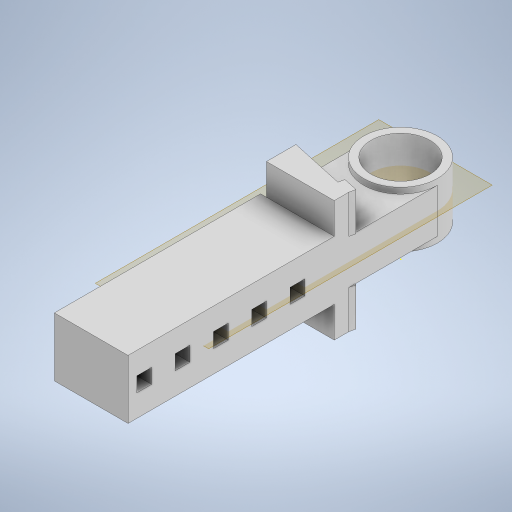
# Autodesk Inventor part: Part10copycopy
Saved by Autodesk Inventor 2023 (Build 270158000, 158)
## iProperties
Created: 2024-11-26
Part Number: Part10copycopy
Material: Generic
Document SubType Name: Modeling
Designer: 1ZHUSAM
Density: 1 g/cm^3
Appearance: Default
Author: 1ZHUSAM
Autodesk Inventor part; units mm, degrees
ref_plane "YZ Plane" through (0, 0, 0) normal (1, 0, 0) x (0, 1, 0)
ref_plane "XY Plane" through (0, 0, 0) normal (0, 0, 1) x (1, 0, 0)
sketch "Sketch1" plane through (0, 0, 0) normal (0, 1, 0) x (-1, 0, 0)
  circle A0 centre (0, 0) radius 10
  circle A1 centre (0, 0) radius 12.5
  line L0 (12.5, 0) -> (12.5, 50)
  line L1 (-12.5, 0) -> (-12.5, 50)
  line L2 (-12.5, 50) -> (12.5, 50)
  dimension "d0" = 20
  dimension "d1" = 25
  dimension "d2" = 50
  constraints: 6 end point, 2 centre point, 2 coincident, 2 point on circle, 2 tangent, 2 vertical, 1 perpendicular
  measures "d0" diameter of A0
  measures "d1" diameter of A1
  measures "d2" distance of L0.start L0.end
extrude "Extrusion1" add sketch "Sketch1" along normal blind 15
sketch "Sketch3" plane through (-12.5, 0, 50) normal (0, 0, 1) x (1, 0, 0)
  point P0 (12.5, 0)
sketch "Sketch4" plane through (-12.5, 0, 50) normal (0, 0, 1) x (1, 0, 0)
  line L0 (25, 0) -> (25, 15) projected
  line L1 (25, 0) -> (25, 15)
  line L2 (0, 15) -> (25, 15) projected
  line L3 (25, 15) -> (0, 15)
  line L4 (0, 0) -> (0, 15) projected
  line L5 (0, 15) -> (0, 0)
  line L6 (0, 0) -> (25, 0) projected
  line L7 (0, 0) -> (25, 0)
  point P0 (12.5, 0)
  constraints: 8 end point, 4 collinear
extrude "Extrusion3" add sketch "Sketch4" along normal blind 25
sketch "Sketch9" plane through (0, 0, 0) normal (0, -1, 0) x (1, 0, 0)
  line L0 (-12.5, 25) -> (-22.5, 25) projected
  line L1 (-12.5, 25) -> (12.5, 25)
  line L2 (12.5, 0) -> (12.5, 75) projected
  line L3 (-12.5, 25) -> (-12.5, 75) projected
  line L4 (-12.5, 25) -> (-12.5, 75)
  line L5 (-12.5, 75) -> (12.5, 75) projected
  line L6 (-12.5, 75) -> (12.5, 75)
  line L7 (12.5, 75) -> (12.5, 25)
  line L8 (12.5, 0) -> (12.5, 30)
  line L9 (-12.5, 25) -> (-10.5, 25)
  line L10 (-10.5, 25) -> (-10.5, 75)
  line L11 (-12.5, 75) -> (-12.5, 25)
  line L12 (-10.5, 25) -> (12.5, 30)
  line L13 (-10.5, 25) -> (-10.5, 35)
  line L14 (-10.5, 35) -> (12.5, 35)
  point P0 (0, 0)
  point P1 (12.5, 35)
  dimension "d50" = 30
  dimension "d51" = 2
  dimension "d74" = 10
  constraints: 22 end point, 7 point on line, 3 collinear, 3 perpendicular, 1 horizontal
  measures "d50" distance of L8.start L8.end
  measures "d51" distance of L0.start L9.end
  measures "d74" distance of L9.end L13.end
extrude "Extrusion7" add sketch "Sketch9" along normal blind 13 contours L10 L14 L2 L12
sketch "Sketch10" plane through (0, -13, 0) normal (0, -1, 0) x (1, 0, 0)
  point P0 (0, 0)
ref_plane "Work Plane1" through (0, 7.5, 0) normal (0, 1, 0) x (-1, 0, 0)
mirror "Mirror1" about plane through (0, 7.5, 0) normal (0, 1, 0) of "Extrusion7"
sketch "Sketch15" plane through (-10.5, 15, 25) normal (0.2124296, 0, -0.9771764) x (-0.9771764, 0, -0.2124296)
  line L0 (-23.5372, 0) -> (-23.5372, 13) projected
  line L1 (-14.7001, 13) -> (-18.6088, 13) projected
  line L2 (-23.5372, 0) -> (-18.5372, 0)
  line L3 (-18.5372, 0) -> (-18.5372, 13)
  line L4 (-18.5372, 13) -> (-23.5372, 13)
  line L5 (-23.5372, 13) -> (-23.5372, 0)
  line L6 (-23.5372, -28) -> (-24.5994, -28) projected
  line L7 (-18.6088, -28) -> (-18.6088, 13) projected
  line L8 (-23.5372, -28) -> (-18.6088, -28)
  line L9 (-18.6088, -28) -> (-18.6088, -15)
  line L10 (-18.6088, -15) -> (-23.5372, -15)
  line L11 (-23.5372, -15) -> (-23.5372, -28)
  point P0 (-4.9496, -15)
  point P1 (-33.0965, -28)
  point P2 (-18.6088, 0)
  point P3 (-23.5372, 13)
  dimension "d66" = 5
  constraints: 16 end point, 4 parallel, 2 horizontal, 2 perpendicular, 2 point on line
  measures "d66" distance of L4.end L3.end
extrude "Extrusion9" add sketch "Sketch15" along normal blind 2 contours L0 L4 L7 L2 | L8 L11 L10 L7
sketch "Sketch16" plane through (0, 15, 0) normal (0, 1, 0) x (1, 0, 0)
  circle A0 centre (0, 0) radius 10
  circle A1 centre (0, 0) radius 12.5
  dimension "d69" = 25
  constraints: 2 centre point, 2 coincident
  measures "d69" diameter of A1
extrude "Extrusion10" add sketch "Sketch16" along normal blind 2
sketch "Sketch17" plane through (0, 0, 0) normal (0, -1, 0) x (1, 0, 0)
  circle A0 centre (0, 0) radius 10
  circle A1 centre (0, 0) radius 10 projected
  circle A2 centre (0, 0) radius 12.5
  constraints: 2 centre point, 2 coincident
extrude "Extrusion11" add sketch "Sketch17" along normal blind 2
sketch "Sketch18" plane through (-12.5, 0, 0) normal (-1, 0, 0) x (0, 0, 1)
  point P0 (0, 0)
sketch "Sketch19" plane through (0, 0, 0) normal (0, -1, 0) x (1, 0, 0)
  line L0 (-12.5, 75) -> (12.5, 75) projected
  line L1 (12.5, 35) -> (-10.5, 35) projected
  line L2 (-12.5, 75) -> (12.5, 75)
  line L3 (12.5, 75) -> (12.5, 35)
  line L4 (12.5, 35) -> (-12.5, 35)
  line L5 (-12.5, 35) -> (-12.5, 75)
  point P0 (0, 0)
  constraints: 8 end point, 2 parallel, 1 horizontal, 1 perpendicular
extrude "Extrusion12" add sketch "Sketch19" along normal blind 2.5
sketch "Sketch20" plane through (0, 15, 0) normal (0, 1, 0) x (1, 0, 0)
  line L0 (12.5, -75) -> (-12.5, -75) projected
  line L1 (12.5, -35) -> (12.5, -75) projected
  line L2 (-12.5, -75) -> (12.5, -75)
  line L3 (12.5, -75) -> (12.5, -35)
  line L4 (12.5, -35) -> (-12.5, -35)
  line L5 (-12.5, -35) -> (-12.5, -75)
  point P0 (0, 0)
  constraints: 8 end point, 2 parallel, 1 horizontal, 1 perpendicular
extrude "Extrusion13" add sketch "Sketch20" along normal blind 2.5
sketch "Sketch21" plane through (-12.5, 0, 75) normal (0, 0, 1) x (1, 0, 0)
  line L0 (25, -2.5) -> (0, -2.5) projected
  line L1 (0, -2.5) -> (25, -2.5)
  line L2 (25, -2.5) -> (25, 17.5)
  line L3 (25, 17.5) -> (0, 17.5)
  line L4 (0, 17.5) -> (0, -2.5)
  point P0 (12.5, 0)
  constraints: 8 end point, 2 parallel, 1 horizontal, 1 perpendicular
extrude "Extrusion14" add sketch "Sketch21" along normal blind 30
sketch "Sketch22" plane through (-12.5, 0, 0) normal (-1, 0, 0) x (0, 0, 1)
  line L0 (35, 15) -> (35, 17.5) projected
  line L1 (35, -2.5) -> (105, -2.5) projected
  line L2 (35, 17.5) -> (45, 17.5)
  line L3 (45, 17.5) -> (45, -2.5)
  line L4 (45, -2.5) -> (35, -2.5)
  line L5 (35, -2.5) -> (35, 17.5)
  line L6 (45, 7.5) -> (50, 7.5)
  line L7 (45, 5) -> (50, 5)
  line L8 (50, 5) -> (50, 10)
  line L9 (50, 10) -> (45, 10)
  line L10 (45, 10) -> (45, 5)
  line L11 (45, 5) -> (50, 10) construction
  line L12 (50, 5) -> (45, 10) construction
  line L13 (50, 7.5) -> (58, 7.5)
  line L14 (63, 5) -> (58, 5)
  line L15 (58, 5) -> (58, 10)
  line L16 (58, 10) -> (63, 10)
  line L17 (63, 10) -> (63, 5)
  line L18 (63, 5) -> (58, 10) construction
  line L19 (58, 5) -> (63, 10) construction
  line L20 (63, 7.5) -> (71, 7.5)
  line L21 (76, 5) -> (71, 5)
  line L22 (71, 5) -> (71, 10)
  line L23 (71, 10) -> (76, 10)
  line L24 (76, 10) -> (76, 5)
  line L25 (76, 5) -> (71, 10) construction
  line L26 (71, 5) -> (76, 10) construction
  line L27 (76, 7.5) -> (84, 7.5)
  line L28 (89, 5) -> (84, 5)
  line L29 (84, 5) -> (84, 10)
  line L30 (84, 10) -> (89, 10)
  line L31 (89, 10) -> (89, 5)
  line L32 (89, 5) -> (84, 10) construction
  line L33 (84, 5) -> (89, 10) construction
  line L34 (89, 7.5) -> (97, 7.5)
  line L35 (102, 5) -> (97, 5)
  line L36 (97, 5) -> (97, 10)
  line L37 (97, 10) -> (102, 10)
  line L38 (102, 10) -> (102, 5)
  line L39 (102, 5) -> (97, 10) construction
  line L40 (97, 5) -> (102, 10) construction
  point P0 (0, 0)
  point P1 (47.5, 7.5)
  point P2 (60.5, 7.5)
  point P3 (73.5, 7.5)
  point P4 (86.5, 7.5)
  point P5 (99.5, 7.5)
  dimension "d81" = 10
  dimension "d82" = 5
  dimension "d83" = 5
  dimension "d84" = 8
  dimension "d85" = 5
  dimension "d86" = 8
  dimension "d87" = 8
  dimension "d88" = 8
  constraints: 78 end point, 15 midpoint, 12 parallel, 11 horizontal, 6 perpendicular, 3 point on line
  measures "d81" distance of L3.end L4.end
  measures "d82" distance of L6.start L6.end
  measures "d83" distance of L8.end L7.end
  measures "d84" distance of L6.end L13.end
  measures "d85" distance of L14.end L15.end
  measures "d86" distance of L20.start L20.end
  measures "d87" distance of L27.start L27.end
  measures "d88" distance of L34.start L34.end
extrude "Extrusion15" cut sketch "Sketch22" against normal blind 30 contours L9 L8 L6 L3 | L3 L6 L8 L7 | L14 L15 L16 L17 | L21 L22 L23 L24 | L28 L29 L30 L31 | L35 L36 L37 L38
body "Solid1"
